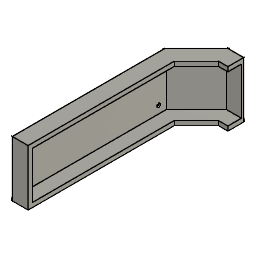
case left v15 (Autodesk Fusion 360 design; units mm, degrees)
Autodesk Fusion 360 part; units mm, degrees
sketch "Sketch1" plane through (0, 0, 0) normal (0, 0, 1) x (1, 0, 0)
  line L0 (0, 0) -> (0, 98) construction
  line L1 (0, 98) -> (20, 118) construction
  line L2 (20, 118) -> (30, 118) construction
  line L3 (9, 0) -> (9, 94.2721)
  line L4 (9, 94.2721) -> (23.7279, 109)
  line L5 (23.7279, 109) -> (30, 109)
  line L6 (-3, 0) -> (-3, 99.2426)
  line L7 (-3, 99.2426) -> (18.7574, 121)
  line L8 (18.7574, 121) -> (30, 121)
  line L9 (0, 0) -> (9, 0) construction
  line L10 (0, 0) -> (-3, 0) construction
  line L11 (30, 118) -> (30, 109)
  line L12 (30, 118) -> (30, 121)
  line L13 (0, -3) -> (9, -3)
  line L14 (0, -3) -> (-3, -3)
  line L15 (9, -3) -> (9, 0)
  line L16 (-3, -3) -> (-3, 0)
  dimension "d7" = 98
  dimension "d8" = 135
  dimension "d9" = 118
  dimension "d10" = 10
  dimension "d11" = 9
  dimension "d12" = -3
  dimension "d13" = 3
  constraint coincident L0.start L9.start
  constraint vertical L0
  constraint perpendicular L0 L2
  constraint perpendicular L3 L9
  constraint perpendicular L6 L10
  constraint perpendicular L5 L11
  constraint perpendicular L8 L12
  constraint perpendicular L9 L15
  constraint perpendicular L10 L16
  measures "d7" distance of L0.start L0.end
  measures "d8" angle of L0 L1
  measures "d9" vertical distance of L0.start L1.end
  measures "d10" distance of L1.end L2.end
extrude "Extrude1" add sketch "Sketch1" along normal blind 37.22
shell "Shell1" thickness 3 removed faces 4 at (30, 119, 12.4067) at (25.8186, 109, 12.4067) at (13.9093, 99.1814, 24.8133) at (9, 31.424, 12.4067)
sketch "Sketch2" plane through (-3, 0, 0) normal (-1, 0, 0) x (0, -1, 0)
  line L0 (-99.2426, 0) -> (3, 0)
  line L1 (3, 0) -> (3, 37.22)
  line L2 (3, 37.22) -> (-99.2426, 37.22)
  line L3 (-99.2426, 37.22) -> (-99.2426, 0)
  line L4 (0, 3) -> (-98, 3) construction
  line L5 (-98, 3) -> (-98, 34.22) construction
  line L6 (-98, 34.22) -> (0, 34.22) construction
  line L7 (0, 34.22) -> (0, 3) construction
  circle A0 centre (-5, 29.22) radius 2
  circle A1 centre (-93, 8) radius 1.3
  circle A2 centre (-93, 8) radius 2
  circle A3 centre (-5, 29.22) radius 1.3
  dimension "d21" = 3
  dimension "d22" = 3
  dimension "d23" = 3
  dimension "d24" = 98
  dimension "d25" = 2.6
  dimension "d26" = 4
  dimension "d27" = 5
  dimension "d28" = 5
  dimension "d29" = 5
  dimension "d30" = 5
  dimension "d31" = 2.6
  dimension "d32" = 4
  constraint horizontal L4
  constraint vertical L5
  constraint horizontal L6
  constraint vertical L7
  constraint concentric A1 A2
  constraint concentric A0 A3
  measures "d21" distance of L0 L4
  measures "d22" distance of L2 L6
  measures "d23" distance of L1 L7
  measures "d24" distance of L5.end L6.end
  measures "d25" diameter of A1
  measures "d26" diameter of A2
  measures "d27" distance of L4 A1.centre
  measures "d28" distance of L5 A1.centre
  measures "d29" distance of L6 A0.centre
  measures "d30" distance of L7 A0.centre
  measures "d31" diameter of A3
  measures "d32" diameter of A0
extrude "Extrude2" cut sketch "Sketch2" against normal through all contours A1 | A3
extrude "Extrude3" cut sketch "Sketch2" against normal blind 2 contours A0 | A2
fillet "Fillet3" radius 1.5 10 edges at (-3, -3, 18.61) (-3, 48.1213, 37.22) (-3, 48.1213, 0) (-3, 99.2426, 18.61) (7.8787, 110.1213, 37.22) (7.8787, 110.1213, 0) (18.7574, 121, 18.61) (24.3787, 121, 37.22) (24.3787, 121, 0) (30, 121, 18.61)
